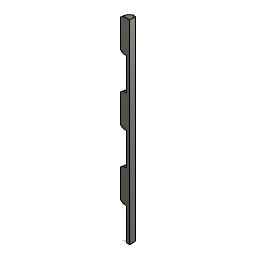
pencil case clasp - alternating wedges v2 (Autodesk Fusion 360 design; units mm, degrees)
Autodesk Fusion 360 part; units mm, degrees
note: some values were not read from the file. Chosen so that the rebuilt part matches the saved one: which bodies a step acts on.
sketch "wedge side" plane through (0, 0, 0) normal (0, 1, 0) x (1, 0, 0)
  line L0 (0, 0) -> (5.0614, 5.0614)
  line L1 (0, 0) -> (7.1578, 0) construction
  line L2 (0, 0) -> (-1.312, -1.312)
  line L3 (-1.312, -1.312) -> (-10.924, -10.924)
  line L4 (12.4749, 3) -> (-4.8473, 3)
  line L5 (8.9736, -3) -> (-11.747, -3)
  line L6 (6, 3) -> (6, -3)
  dimension "d3" = 45
  dimension "d4" = 3
  dimension "d5" = 3
  dimension "d6" = 6
  constraint horizontal L1
  constraint coincident L0.start L1.start
  constraint parallel L0 L2
  constraint parallel L0 L3
  constraint horizontal L4
  constraint horizontal L5
  constraint coincident L4 L6.start
  constraint coincident L5 L6.end
  constraint perpendicular L5 L6
  measures "d3" angle of L0 L1
  measures "d4" distance of L0.start L4
  measures "d5" distance of L0.start L5
  measures "d6" distance of L0.start L6
extrude "Extrude1" add sketch "wedge side" along normal blind 33 makes body 1
sketch "clip corners" plane through (0, 0, 3) normal (0, 0, 1) x (1, 0, 0)
  line L0 (-3, 0) -> (6, 0)
  line L1 (6, 0) -> (6, 33)
  line L2 (6, 33) -> (-3, 33)
  line L3 (-3, 33) -> (-3, 0)
  line L4 (-3, 31) -> (0, 33)
  line L5 (6, 16.5) -> (-3, 16.5) construction
  line L6 (-3, 2) -> (0, 0)
  dimension "d9" = 2
  dimension "d10" = 3
  constraint coincident L3 L4.start
  constraint coincident L2 L4.end
  constraint midpoint L1 L5.start
  constraint midpoint L3 L5.end
  constraint symmetric L4.start L5 L6.start
  constraint symmetric L4.end L5 L6.end
  measures "d9" distance of L2.end L4.start
  measures "d10" distance of L2.end L4.end
extrude "Extrude2" cut sketch "clip corners" against normal blind 10 contours L0 L3 L6 | L2 L3 L4 bodies 1
copy_body "CopyPasteBodies1" bodies 1 makes body 2
move_body "Move1" bodies 2 to x (1, 0, 0) y (0, -1, 0) z (0, 0, -1) at (0, 0, 0)
combine "Combine1" operation add target body 1 tool bodies 2
pattern_linear "R-Pattern1" count 3 spacing 66 along (0, 1, 0) both ways of bodies 1 makes body 3 at (6, 55, -1) makes body 4 at (6, -77, -1)
combine "Combine2" operation add target body 1 tool bodies 3 4
named bodies: "pencil case clasp top", "pencil case clasp top (1)"
